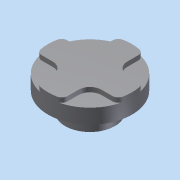
# Autodesk Inventor part: XBox360DirectionalPad
Saved by Autodesk Inventor 2011 SP1 (Build 150282100, 282)
## iProperties
Created: 2011-08-14
Part Number: XBox360DirectionalPad
Document SubType Name: Modeling
Designer: dgitz
Density: 1 g/cm^3
Author: dgitz
Autodesk Inventor part; units mm, degrees
ref_plane "YZ Plane" through (0, 0, 0) normal (1, 0, 0) x (0, 1, 0)
ref_plane "XZ Plane" through (0, 0, 0) normal (0, 1, 0) x (-1, 0, 0)
ref_plane "XY Plane" through (0, 0, 0) normal (0, 0, 1) x (1, 0, 0)
sketch "Sketch1" plane through (0, 0, 0) normal (0, 0, 1) x (1, 0, 0)
  point P0 (0, 0)
sketch "Sketch2" plane through (0, 0, 0) normal (0, 1, 0) x (-1, 0, 0)
  circle A0 centre (0, 0) radius 11.557
  dimension "d0" = 23.114
  constraints: 1 centre point, 1 coincident
  measures "d0" diameter of A0
extrude "Extrusion1" add sketch "Sketch2" along normal blind 4.064
sketch "Sketch5" plane through (0, 4.064, 0) normal (0, 1, 0) x (1, 0, 0)
  circle A0 centre (0, 0) radius 11.557 projected
  arc A1 (2.282, 11.3295) -> (-2.282, 11.3295) centre (0, 0) ccw
  arc A2 (11.3295, -2.282) -> (11.3295, 2.282) centre (0, 0) ccw
  arc A3 (-11.3295, 2.282) -> (-11.3295, -2.282) centre (0, 0) ccw
  arc A4 (-2.282, -11.3295) -> (2.282, -11.3295) centre (0, 0) ccw
  line L0 (-3.556, 9.7732) -> (-3.556, 6.731)
  line L1 (-3.556, -6.731) -> (-3.556, -9.7732)
  line L2 (-9.7732, -3.556) -> (-6.731, -3.556)
  line L3 (6.731, -3.556) -> (9.7732, -3.556)
  line L4 (3.556, 9.7732) -> (3.556, 6.731)
  line L5 (3.556, -6.731) -> (3.556, -9.7732)
  line L6 (-9.7732, 3.556) -> (-6.731, 3.556)
  line L7 (6.731, 3.556) -> (9.7732, 3.556)
  arc A5 (-6.731, 3.556) -> (-3.556, 6.731) centre (-6.731, 6.731) ccw
  arc A6 (-3.556, -6.731) -> (-6.731, -3.556) centre (-6.731, -6.731) ccw
  arc A7 (6.731, -3.556) -> (3.556, -6.731) centre (6.731, -6.731) ccw
  arc A8 (3.556, 6.731) -> (6.731, 3.556) centre (6.731, 6.731) ccw
  arc A9 (-2.282, 11.3295) -> (-3.556, 9.7732) centre (-1.9685, 9.7732) ccw
  arc A10 (3.556, 9.7732) -> (2.282, 11.3295) centre (1.9685, 9.7732) ccw
  arc A11 (11.3295, 2.282) -> (9.7732, 3.556) centre (9.7732, 1.9685) ccw
  arc A12 (9.7732, -3.556) -> (11.3295, -2.282) centre (9.7732, -1.9685) ccw
  arc A13 (2.282, -11.3295) -> (3.556, -9.7732) centre (1.9685, -9.7732) ccw
  arc A14 (-3.556, -9.7732) -> (-2.282, -11.3295) centre (-1.9685, -9.7732) ccw
  arc A15 (-11.3295, -2.282) -> (-9.7732, -3.556) centre (-9.7732, -1.9685) ccw
  arc A16 (-9.7732, 3.556) -> (-11.3295, 2.282) centre (-9.7732, 1.9685) ccw
  point P0 (-3.556, 10.9963)
  point P1 (-3.556, -10.9963)
  point P2 (3.556, 10.9963)
  point P3 (3.556, -10.9963)
  point P4 (-10.9963, 3.556)
  point P5 (10.9963, 3.556)
  point P6 (-10.9963, -3.556)
  point P7 (10.9963, -3.556)
  dimension "d23" = 3.175
  dimension "d24" = 1.5875
  constraints: 40 point on circle, 24 tangent, 16 centre point, 16 end point, 10 equal radius, 8 parallel, 8 point on line, 4 perpendicular, 2 vertical, 1 coincident
  measures "d23" radius of A5
  measures "d24" radius of A9
extrude "Extrusion2" add sketch "Sketch5" along normal blind 1.27 contours A0 A12 L3 A7 L5 A13 A14 L1 A6 L2 A15 A16 L6 A5 L0 A9 A10 L4 A8 L7 A11
sketch "Sketch6" plane through (0, 0, 0) normal (0, -1, 0) x (1, 0, 0)
  circle A0 centre (0, 0) radius 11.557 projected
  circle A1 centre (0, 0) radius 6.858
  dimension "d27" = 13.716
  constraints: 1 centre point, 1 coincident
  measures "d27" diameter of A1
extrude "Extrusion3" add sketch "Sketch6" along normal blind 5.08 contours A1
body "Solid1"
